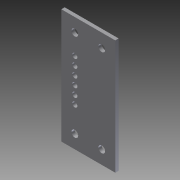
# Autodesk Inventor part: AS2-8-4-001
Saved by Autodesk Inventor 2011 SP1 (Build 150282100, 282)
## iProperties
Created: 2011-01-12
Part Number: AS2-8-4-001
Document SubType Name: Modeling
Designer: Christopher
Density: 1 g/cm^3
Author: Christopher
Autodesk Inventor part; units mm, degrees
ref_plane "YZ Plane" through (0, 0, 0) normal (1, 0, 0) x (0, 1, 0)
ref_plane "XZ Plane" through (0, 0, 0) normal (0, 1, 0) x (-1, 0, 0)
ref_plane "XY Plane" through (0, 0, 0) normal (0, 0, 1) x (1, 0, 0)
sketch "Sketch1" plane through (0, 0, 0) normal (0, 0, 1) x (1, 0, 0)
  line L0 (-20.7908, 24.2777) -> (30.0092, 24.2777)
  line L1 (30.0092, 24.2777) -> (30.0092, -83.6723)
  line L2 (30.0092, -83.6723) -> (-20.7908, -83.6723)
  line L3 (-20.7908, -83.6723) -> (-20.7908, 24.2777)
  line L4 (26.8342, 24.2777) -> (26.8342, -1.1223)
  line L5 (26.8342, -1.1223) -> (30.0092, -1.1223)
  line L6 (26.8342, -83.6723) -> (26.8342, -58.2723)
  line L7 (26.8342, -58.2723) -> (30.0092, -58.2723)
  point P0 (0, 0)
  point P1 (-8.0908, 11.5777)
  point P2 (17.3092, 11.5777)
  point P3 (-8.0908, -70.9723)
  point P4 (17.3092, -70.9723)
  point P5 (-8.0908, -7.4723)
  point P6 (-8.0908, -15.4098)
  point P7 (-8.0908, -23.3473)
  point P8 (-8.0908, -31.2848)
  point P9 (-8.0908, -39.2223)
  point P10 (-8.0908, -47.1598)
  dimension "d0" = 50.8
  dimension "d1" = 107.95
  dimension "d2" = 12.7
  dimension "d3" = 12.7
  dimension "d4" = 12.7
  dimension "d5" = 12.7
  dimension "d6" = 12.7
  dimension "d7" = 12.7
  dimension "d8" = 12.7
  dimension "d9" = 12.7
  dimension "d12" = 7.9375
  dimension "d13" = 7.9375
  dimension "d14" = 7.9375
  dimension "d15" = 7.9375
  dimension "d16" = 7.9375
  dimension "d36" = 38.1
  dimension "d37" = 38.1
  dimension "d38" = 38.1
  dimension "d39" = 38.1
  dimension "d40" = 19.05
  dimension "d41" = 38.1
  dimension "d43" = 38.1
  dimension "d44" = 25.4
  dimension "d45" = 3.175
  dimension "d46" = 25.4
  dimension "d47" = 3.175
  constraints: 16 end point, 4 parallel, 4 point on line, 3 perpendicular, 1 horizontal
  measures "d0" distance of L0.start L0.end
  measures "d1" distance of L2.end L0.start
  measures "d2" distance from line of L0 point (-8.091, 11.578)
  measures "d3" distance from line of L3 point (-8.091, 11.578)
  measures "d4" distance from line of L0 point (17.309, 11.578)
  measures "d5" distance from line of L1 point (17.309, 11.578)
  measures "d6" distance from line of L2 point (-8.091, -70.972)
  measures "d7" distance from line of L2 point (17.309, -70.972)
  measures "d8" distance from line of L1 point (17.309, -70.972)
  measures "d9" distance from line of L3 point (-8.091, -70.972)
  measures "d12" distance of point (-8.091, -7.472) point (-8.091, -15.41)
  measures "d13" distance of point (-8.091, -15.41) point (-8.091, -23.347)
  measures "d14" distance of point (-8.091, -23.347) point (-8.091, -31.285)
  measures "d15" distance of point (-8.091, -31.285) point (-8.091, -39.222)
  measures "d16" distance of point (-8.091, -39.222) point (-8.091, -47.16)
  measures "d36" distance from line of L1 point (-8.091, -7.472)
  measures "d37" distance from line of L1 point (-8.091, -15.41)
  measures "d38" distance from line of L1 point (-8.091, -23.347)
  measures "d39" distance from line of L1 point (-8.091, -31.285)
  measures "d40" distance of point (-8.091, 11.578) point (-8.091, -7.472)
  measures "d41" distance from line of L1 point (-8.091, -39.222)
  measures "d43" distance from line of L1 point (-8.091, -47.16)
  measures "d44" distance of L6.start L6.end
  measures "d45" distance of L6.end L7.end
  measures "d46" distance of L4.start L4.end
  measures "d47" distance of L4.end L5.end
extrude "Extrusion1" add sketch "Sketch1" against normal blind 3.175
hole "Hole1" at (-8.0908, 11.5777, 0) at (17.3092, 11.5777, 0) at (-8.0908, -70.9723, 0) at (17.3092, -70.9723, 0) direction (0, 0, -1) diameter 6.35 depth 25.4 tip angle 118
hole "Hole2" at (-8.0908, -7.4723, 0) at (-8.0908, -15.4098, 0) at (-8.0908, -23.3473, 0) at (-8.0908, -31.2848, 0) at (-8.0908, -39.2223, 0) at (-8.0908, -47.1598, 0) direction (0, 0, -1) diameter 4.7625 depth 25.4 tip angle 118
body "Solid1"
